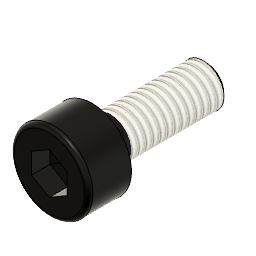
Hexagon Socket Head Cap Screw DIN 912 - M3 x 0.5 x 8 Steel 4.6 Black (Autodesk Fusion 360 design; units mm, degrees)
description: Hexagon Socket Head Cap Screw DIN 912 - M3 x 0.5 x 8
part number: DIN 912 - M3 x 0.5 x 8 Steel 4.6 Black
Autodesk Fusion 360 part; units mm, degrees
sketch "Sketch1" plane through (0, 0, 0) normal (0, 1, 0) x (1, 0, 0)
  line L0 (-1.5, 0) -> (-1.5, 8)
  line L1 (-1.5, 8) -> (0, 8)
  line L2 (0, 8) -> (0, -3)
  line L3 (-1.5, 0) -> (-2.75, 0)
  line L4 (-2.75, 0) -> (-2.75, -3)
  line L5 (-2.75, -3) -> (0, -3)
  dimension "d101" = 8
  dimension "d102" = 3
  dimension "d109" = 5.5
  dimension "d110" = 3
  constraint perpendicular L0 L1
  constraint collinear origin L1.end L2.end
  constraint perpendicular L0 L3
  constraint coincident origin L3
  constraint vertical L2
  constraint coincident L2 L5.end
  constraint perpendicular L2 L5
  measures "d101" distance of origin L1
  measures "d102" distance of L3.end L5
revolve "Revolve1" add sketch "Sketch1" angle 360 about axis through (0, 0, -8) along (0, 0, 1)
ref_plane "WorkPlane1" through (0, 0, 3) normal (0, 0, 1) x (1, 0, 0)
sketch "Sketch6" plane through (0, 0, 3) normal (0, 0, 1) x (1, 0, 0)
  line L0 (0, -1.4434) -> (1.25, -0.7217)
  line L1 (1.25, -0.7217) -> (1.25, 0.7217)
  line L2 (1.25, 0.7217) -> (0, 1.4434)
  line L3 (0, 1.4434) -> (-1.25, 0.7217)
  line L4 (-1.25, 0.7217) -> (-1.25, -0.7217)
  line L5 (-1.25, -0.7217) -> (0, -1.4434)
  dimension "d111" = 2.5
  constraint vertical L1
  measures "d111" distance of L1 L4
extrude "Extrude1" cut sketch "Sketch6" against normal blind 1.3
extrude "Extrude2" cut 1 faces at (0.4167, -0.2406, 1.7) along direction (0, 0, -1) blind 1.3 draft -85
thread "Thread3" "ISO Metric profile 3.0 M3x0.5 M3x0.5 6g" major diameter 2.927 minor diameter 2.3555 pitch 0.5 angle 60 resizes the face on face at (-1.4925, 0.1494, -5.3333) from (0, 0, -1.25) to (0, 0, -8)
fillet "Fillet4" radius 0.3 1 edges at (-2.5639, 0.9944, 3)
sketch "Sketch7" plane through (0, 0, 0) normal (0, 1, 0) x (1, 0, 0)
  line L0 (-1.53, 8) -> (-1.53, 7.6933)
  line L1 (-1.53, 7.6933) -> (-1.1933, 8)
  line L2 (0, 8) -> (0, -3)
  line L3 (-1.53, 8) -> (0, 8)
  dimension "d104" = 1.1933
  dimension "d105" = 1.53
  dimension "d106" = 0.3067
  constraint coincident L2.start L3.end
  constraint perpendicular L2 L3
  constraint coincident L1.end L3
  constraint perpendicular L0 L3
  measures "d104" distance of L1.end L2
  measures "d105" distance of L0 L2.start
  measures "d106" distance of L0.end L3
revolve "Revolve3" cut sketch "Sketch7" angle 360 about axis through (0, 0, 1.75) along (0, 0, 1)
equation "adsk_nomlen = 8.00 mm"
equation "adsk_headh = 3.00 mm"
equation "adsk_headdia = 5.50 mm"
equation "adsk_nomdia = 3.00 mm"
equation "adsk_philwidth = 2.50 mm"
equation "d31 = -adsk_phildepth"
equation "adsk_phildepth = 1.30 mm"
equation "d71 = adsk_headh"
equation "d76 = -adsk_phildepth"
equation "adsk_thrlen = 6.75 mm"
equation "d86 = adsk_nomdia * 0.1"
equation "adsk_startlen = 0.306725 mm"
equation "adsk_endpointdia = 2.38655 mm"
equation "d101 = adsk_nomlen"
equation "d102 = adsk_headh"
equation "d104 = adsk_endpointdia / 2"
equation "d105 = adsk_nomdia * 0.51"
equation "d106 = adsk_startlen"
equation "d108 = min(adsk_thrlen; adsk_nomlen - 0.001 mm)"
equation "d109 = adsk_headdia"
equation "d110 = adsk_nomdia"
equation "d111 = adsk_philwidth"
